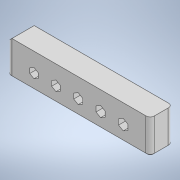
# Autodesk Inventor part: Тестер втулок
Saved by Autodesk Inventor 2021.2 (Build 252289000, 289)
## iProperties
Created: 2024-11-21
Part Number: Тестер втулок
Material: Типовые
Document SubType Name: Modeling
Designer: Barcock
Density: 1 g/cm^3
Appearance: По умолчанию
Author: Barcock
Autodesk Inventor part; units mm, degrees
ref_plane "YZ Plane" through (0, 0, 0) normal (1, 0, 0) x (0, 1, 0)
ref_plane "XZ Plane" through (0, 0, 0) normal (0, 1, 0) x (-1, 0, 0)
ref_plane "XY Plane" through (0, 0, 0) normal (0, 0, 1) x (1, 0, 0)
sketch "Эскиз2" plane through (0, 0, 0) normal (0, 0, 1) x (1, 0, 0)
  circle A0 centre (11.9, 0) radius 1.9 construction
  line L0 (0, 0) -> (64, 0) construction
  line L1 (11.9, -2.1939) -> (10, -1.097)
  line L2 (10, -1.097) -> (10, 1.097)
  line L3 (10, 1.097) -> (11.9, 2.1939)
  line L4 (11.9, 2.1939) -> (13.8, 1.097)
  line L5 (13.8, 1.097) -> (13.8, -1.097)
  line L6 (13.8, -1.097) -> (11.9, -2.1939)
  circle A1 centre (21.75, 0) radius 1.95 construction
  circle A2 centre (31.7, 0) radius 2 construction
  circle A3 centre (41.75, 0) radius 2.05 construction
  circle A4 centre (51.9, 0) radius 2.1 construction
  line L7 (21.75, -2.2517) -> (19.8, -1.1258)
  line L8 (19.8, -1.1258) -> (19.8, 1.1258)
  line L9 (19.8, 1.1258) -> (21.75, 2.2517)
  line L10 (21.75, 2.2517) -> (23.7, 1.1258)
  line L11 (23.7, 1.1258) -> (23.7, -1.1258)
  line L12 (23.7, -1.1258) -> (21.75, -2.2517)
  line L13 (31.7, -2.3094) -> (29.7, -1.1547)
  line L14 (29.7, -1.1547) -> (29.7, 1.1547)
  line L15 (29.7, 1.1547) -> (31.7, 2.3094)
  line L16 (31.7, 2.3094) -> (33.7, 1.1547)
  line L17 (33.7, 1.1547) -> (33.7, -1.1547)
  line L18 (33.7, -1.1547) -> (31.7, -2.3094)
  line L19 (41.75, -2.3671) -> (39.7, -1.1836)
  line L20 (39.7, -1.1836) -> (39.7, 1.1836)
  line L21 (39.7, 1.1836) -> (41.75, 2.3671)
  line L22 (41.75, 2.3671) -> (43.8, 1.1836)
  line L23 (43.8, 1.1836) -> (43.8, -1.1836)
  line L24 (43.8, -1.1836) -> (41.75, -2.3671)
  line L25 (51.9, -2.4249) -> (49.8, -1.2124)
  line L26 (49.8, -1.2124) -> (49.8, 1.2124)
  line L27 (49.8, 1.2124) -> (51.9, 2.4249)
  line L28 (51.9, 2.4249) -> (54, 1.2124)
  line L29 (54, 1.2124) -> (54, -1.2124)
  line L30 (54, -1.2124) -> (51.9, -2.4249)
  line L31 (2, 8.5) -> (64, 8.5)
  line L32 (64, 8.5) -> (64, -6.5)
  line L33 (64, -6.5) -> (0, -6.5)
  line L34 (0, -6.5) -> (0, 6.5)
  line L35 (0, 6.5) -> (2, 8.5)
  point P0 (11.9, 0)
  point P1 (21.75, 0)
  point P2 (41.75, 0)
  point P3 (51.9, 0)
  point P4 (0, 8.5)
  dimension "d3" = 6
  dimension "d4" = 6
  dimension "d5" = 6
  dimension "d6" = 6
  dimension "d7" = 15
  dimension "d8" = 10
  dimension "d9" = 10
  dimension "d10" = 3.8
  dimension "d11" = 3.9
  dimension "d12" = 4
  dimension "d13" = 4.1
  dimension "d14" = 4.2
  dimension "d15" = 2
  dimension "d16" = 2
  constraints: 72 end point, 8 point on line, 5 centre point, 5 coincident, 5 tangent, 5 vertical, 2 horizontal, 2 parallel, 1 midpoint, 1 perpendicular, 65 other
  measures "d3" distance between parallel lines of L5 L8
  measures "d4" distance between parallel lines of L14 L11
  measures "d5" distance between parallel lines of L23 L26
  measures "d6" distance between parallel lines of L17 L20
  measures "d7" distance of L33.end point (0, 8.5)
  measures "d8" distance between parallel lines of L32 L29
  measures "d9" distance between parallel lines of L34 L2
  measures "d10" diameter of A0
  measures "d11" diameter of A1
  measures "d12" diameter of A2
  measures "d13" diameter of A3
  measures "d14" diameter of A4
  measures "d15" distance of L34.end point (0, 8.5)
  measures "d16" distance of L31.start point (0, 8.5)
extrude "Выдавливание2" add sketch "Эскиз2" along normal blind 10
fillet "Сопряжение1" radius 2 4 edges at (0, 0, 10) (0, 0, 0) (64, 1, 0) (64, 1, 10) curvature continuous yes
chamfer "Фаска1" distance 0.5 angle 45 8 edges at (32, -6.5, 10) (63.4819, -6.5, 9.4822) (64, -6.5, 5) (63.4819, -6.5, 0.5178) (32, -6.5, 0) (0.5179, -6.5, 0.518) (0, -6.5, 5) (0.5181, -6.5, 9.4822)
equation "\"d4\" = d3"
equation "\"d5\" = d6"
equation "\"d6\" = d4"
equation "\"d16\" = d15"
